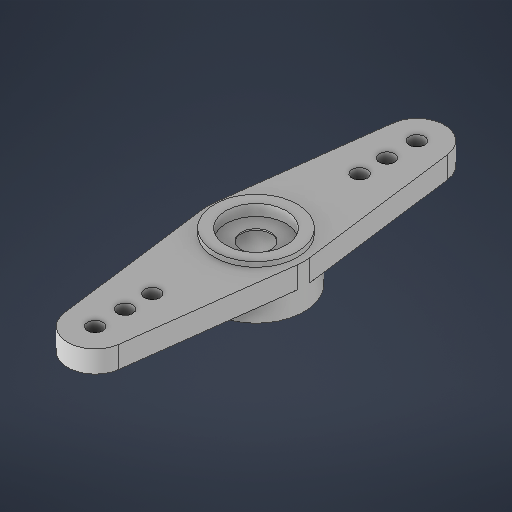
# Autodesk Inventor part: MMAE 232 CAD Assignment 2 Servo Horn 6-Nicholas Skiba
Saved by Autodesk Inventor 2026.1 (Build 301233000, 233)
## iProperties
Created: 2025-08-27
Part Number: MMAE 232 CAD Assignment 2 Servo Horn 6-Nicholas Skiba
Material: Generic
Document SubType Name: Modeling
Designer: Nick
Density: 1 g/cm^3
Appearance: Default
Author: Nick
Autodesk Inventor part; units mm, degrees
ref_plane "YZ Plane" through (0, 0, 0) normal (1, 0, 0) x (0, 1, 0)
ref_plane "XZ Plane" through (0, 0, 0) normal (0, 1, 0) x (-1, 0, 0)
ref_plane "XY Plane" through (0, 0, 0) normal (0, 0, 1) x (1, 0, 0)
sketch "Sketch1" plane through (0, 0, 0) normal (0, 1, 0) x (-1, 0, 0)
  circle A0 centre (0, 0) radius 4.4
  line L0 (9.1763, 0) -> (-11.3805, 0)
  line L1 (0, 0) -> (0, -9.5)
  line L2 (0, -9.5) -> (0, -12)
  line L3 (0, -12) -> (0, -14.74)
  circle A1 centre (0, -9.5) radius 0.7
  circle A2 centre (0, -12) radius 0.7
  circle A3 centre (0, -14.74) radius 0.7
  arc A4 (-2.4994, -15.0614) -> (2.4994, -15.0614) centre (0, -14.74) ccw
  line L4 (2.4994, -15.0614) -> (4.3641, -0.5612)
  line L5 (-2.4994, -15.0614) -> (-4.3641, -0.5612)
  line L6 (0, 0) -> (0, 9.5)
  line L7 (0, 9.5) -> (0, 12)
  line L8 (0, 12) -> (0, 14.74)
  circle A5 centre (0, 9.5) radius 0.7
  circle A6 centre (0, 12) radius 0.7
  circle A7 centre (0, 14.74) radius 0.7
  arc A8 (2.4994, 15.0614) -> (-2.4994, 15.0614) centre (0, 14.74) ccw
  line L9 (2.4994, 15.0614) -> (4.3641, 0.5612)
  line L10 (-2.4994, 15.0614) -> (-4.3641, 0.5612)
  point P0 (4.3641, 0.5612)
  dimension "d0" = 8.8
  dimension "d2" = 9.5
  dimension "d3" = 2.5
  dimension "d4" = 2.74
  dimension "d5" = 1.4
  dimension "d6" = 1.4
  dimension "d7" = 1.4
  dimension "d8" = 5.04
  constraints: 22 end point, 11 symmetric about line, 10 coincident, 9 centre point, 6 point on circle, 4 point on line, 4 tangent, 1 horizontal, 1 vertical, 4 other
  measures "d0" diameter of A0
  measures "d2" distance of L1.start L1.end
  measures "d3" distance of L1.end L2.end
  measures "d4" distance of L2.end L3.end
  measures "d5" diameter of A1
  measures "d6" diameter of A2
  measures "d7" diameter of A3
  measures "d8" diameter of A4
extrude "Extrusion1" add sketch "Sketch1" against normal blind 2 contours A0 L10 A8 L9 | L4 A4 L5 A0
extrude "Extrusion2" add sketch "Sketch1" against normal blind 4 contours L0 L6 A0 | A0 L1 L0 | L1 A0 L0 | L0 A0 L6
sketch "Sketch2" plane through (0, 0, 0) normal (0, 1, 0) x (1, 0, 0)
  circle A0 centre (0, 0) radius 3.785
  circle A1 centre (0, 0) radius 2.75
  dimension "d13" = 7.57
  dimension "d14" = 5.5
  constraints: 2 centre point, 2 coincident
  measures "d13" diameter of A0
  measures "d14" diameter of A1
extrude "Extrusion3" add sketch "Sketch2" along normal blind 0.45
extrude "Extrusion4" cut sketch "Sketch2" against normal blind 0.58 contours A1
sketch "Sketch3" plane through (0, -4, 0) normal (0, -1, 0) x (1, 0, 0)
  circle A0 centre (0, 0) radius 2.75
  circle A1 centre (0, 0) radius 1.375
  dimension "d19" = 5.5
  dimension "d20" = 2.75
  constraints: 2 centre point, 2 coincident
  measures "d19" diameter of A0
  measures "d20" diameter of A1
extrude "Extrusion5" cut sketch "Sketch3" against normal through all contours A1
extrude "Extrusion6" cut sketch "Sketch3" against normal blind 3.3
body "Solid1"
